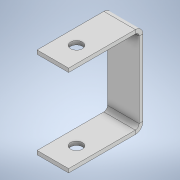
# Autodesk Inventor part: 6x1 BENT
Saved by Autodesk Inventor 2020 (Build 240168000, 168)
## iProperties
Created: 2020-01-01
Part Number: 6x1 BENT
Material: Generic
Document SubType Name: Sheet Metal
Designer: ellio
Density: 1 g/cm^3
Sheet Metal Rule: Default
Appearance: Default
Author: ellio
Autodesk Inventor part; units mm, degrees
ref_plane "YZ Plane" through (0, 0, 0) normal (1, 0, 0) x (0, 1, 0)
ref_plane "XZ Plane" through (0, 0, 0) normal (0, 1, 0) x (-1, 0, 0)
ref_plane "XY Plane" through (0, 0, 0) normal (0, 0, 1) x (1, 0, 0)
sketch "Sketch6" plane through (0, 0, 0) normal (0, 1, 0) x (-1, 0, 0)
  line L0 (0, 0) -> (25.4, 0)
  line L1 (25.4, 0) -> (25.4, -182.118)
  line L2 (25.4, -182.118) -> (0, -182.118)
  line L3 (0, -182.118) -> (0, 0)
  dimension "d32" = 25.4
  dimension "d33" = 182.118
  measures "d32" distance of L1.end L2.end
  measures "d33" distance of L0.end L1.end
extrude "Plate2" add sketch "Sketch6" along normal blind 3.048
sketch "Sketch7" plane through (0, 3.048, 0) normal (0, 1, 0) x (1, 0, 0)
  circle A0 centre (-12.7, 19.05) radius 4.7625
  point P0 (0, 0)
  dimension "d35" = 9.525
  constraints: 1 centre point
  measures "d35" diameter of A0
hole "Hole3" at (-12.7, 3.048, -19.05) direction (0, -1, 0) diameter 9.525 end through all
sketch "Sketch8" plane through (0, 3.048, 0) normal (0, 1, 0) x (1, 0, 0)
  circle A0 centre (-12.7, 163.068) radius 4.7625
  point P0 (0, 0)
  dimension "d43" = 9.525
  constraints: 1 centre point
  measures "d43" diameter of A0
hole "Hole4" at (-12.7, 3.048, -163.068) direction (0, -1, 0) diameter 9.525 end through all
sketch "Sketch9" plane through (0, 3.048, 0) normal (0, 1, 0) x (1, 0, 0)
  line L0 (-25.4, 0) -> (-25.4, 182.118) projected
  line L1 (-25.4, 57.15) -> (0, 57.15)
  point P0 (0, 0)
  constraints: 2 end point, 1 perpendicular, 1 point on line
fold "Fold3" angle 90 bend radius 3.048 thickness 3.048 k factor 0.44 line from (-25.4, 3.048, -57.15) to (0, 3.048, -57.15) line at bend centre moving side (0, 0, -1) folds toward (0, 1, 0)
sketch "Sketch10" plane through (-25.4, 127.6168, -56.7508) normal (0, 0, 1) x (1, 0, 0)
  line L0 (0, -121.5208) -> (0, 0) projected
  line L1 (0, -57.15) -> (25.4, -57.15)
  line L2 (25.4, 0) -> (25.4, -121.5208) projected
  point P0 (25.4, -127.6168)
  constraints: 2 end point, 2 point on line, 1 horizontal
fold "Fold4" angle 90 bend radius 3.048 thickness 3.048 k factor 0.44 line from (-25.4, 70.4668, -56.7508) to (0, 70.4668, -56.7508) line at bend centre moving side (0, 1, 0) folds toward (0, 0, 1)
equation "\"d41\" = Thickness"
equation "\"d49\" = Thickness"
equation "\"d34\" = Thickness"
equation "\"d51\" = BendReliefWidth"
equation "\"d52\" = BendReliefDepth"
equation "\"d53\" = MinimumRemnant"
equation "\"d54\" = TransitionRadius"
equation "\"d56\" = BendRadius"
equation "\"d57\" = BendReliefWidth"
equation "\"d58\" = BendReliefDepth"
equation "\"d59\" = MinimumRemnant"
equation "\"d60\" = TransitionRadius"
equation "\"d62\" = BendRadius"
equation "\"BendRadius\" = Thickness"
equation "\"BendReliefWidth\" = Thickness"
equation "\"BendReliefDepth\" = 0.5 * Thickness"
equation "\"CornerReliefSize\" = 4 * Thickness"
equation "\"MinimumRemnant\" = 2 * Thickness"
equation "\"TransitionRadius\" = BendRadius"
equation "\"JacobiRadiusSize\" = BendRadius"
equation "\"GapSize\" = Thickness"
equation "\"Thickness\" = 3.048"
body "Solid2"
